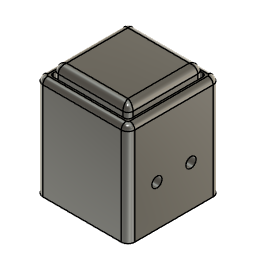
Z_LimitSwitchBox (Autodesk Fusion 360 design; units mm, degrees)
Autodesk Fusion 360 part; units mm, degrees
sketch "Sketch1" plane through (0, 0, 0) normal (0, 0, 1) x (1, 0, 0)
  line L0 (12.5, -12.5) -> (-12.5, -12.5)
  line L1 (-12.5, -12.5) -> (-12.5, 12.5)
  line L2 (-12.5, 12.5) -> (12.5, 12.5)
  line L3 (12.5, 12.5) -> (12.5, -12.5)
  line L4 (12.5, -12.5) -> (-12.5, 12.5) construction
  line L5 (-12.5, -12.5) -> (12.5, 12.5) construction
  line L6 (3.5, -10.5) -> (-3.5, -10.5)
  line L7 (-3.5, -10.5) -> (-3.5, 10.5)
  line L8 (-3.5, 10.5) -> (3.5, 10.5)
  line L9 (3.5, 10.5) -> (3.5, -10.5)
  line L10 (3.5, -10.5) -> (-3.5, 10.5) construction
  line L11 (-3.5, -10.5) -> (3.5, 10.5) construction
  line L12 (11.5, -11.5) -> (-11.5, -11.5)
  line L13 (-11.5, -11.5) -> (-11.5, 11.5)
  line L14 (-11.5, 11.5) -> (11.5, 11.5)
  line L15 (11.5, 11.5) -> (11.5, -11.5)
  line L16 (11.5, -11.5) -> (-11.5, 11.5) construction
  line L17 (-11.5, -11.5) -> (11.5, 11.5) construction
  dimension "d1" = 25
  dimension "d2" = 25
  dimension "d3" = 7
  dimension "d4" = 21
  dimension "d5" = 23
  dimension "d6" = 23
  constraint horizontal L0
  constraint perpendicular L0 L1
  constraint parallel L0 L2
  constraint parallel L1 L3
  constraint coincident L4 origin
  constraint coincident L5 origin
  constraint horizontal L6
  constraint perpendicular L6 L7
  constraint parallel L6 L8
  constraint parallel L7 L9
  constraint coincident L10 origin
  constraint coincident L11 origin
  constraint horizontal L12
  constraint perpendicular L12 L13
  constraint parallel L12 L14
  constraint parallel L13 L15
  constraint coincident L16 origin
  constraint coincident L17 origin
  measures "d1" distance of L1.end L2.end
  measures "d2" distance of L0.end L1.end
  measures "d3" distance of L7.end L8.end
  measures "d4" distance of L6.end L7.end
  measures "d5" distance of L13.end L14.end
  measures "d6" distance of L12.end L13.end
extrude "Extrude1" add sketch "Sketch1" along normal blind 30 contours L0 L1 L2 L3 | L6 L7 L8 L9 | L12 L13 L14 L15 makes body 1
extrude "Extrude2" cut sketch "Sketch1" along normal blind 1000 from surface at 5 contours L6 L7 L8 L9 bodies 1
extrude "Extrude3" cut sketch "Sketch1" along normal blind 100 from surface at 20 contours L12 L13 L14 L15 bodies 1
sketch "Sketch2" plane through (-12.5, 0, 0) normal (-1, 0, 0) x (0, -1, 0)
  line L0 (-12.5, 0) -> (12.5, 0)
  line L1 (12.5, 0) -> (12.5, 30)
  line L2 (12.5, 30) -> (-12.5, 30)
  line L3 (-12.5, 30) -> (-12.5, 0)
  line L4 (0, 12) -> (5, 12)
  line L5 (0, 12) -> (-5, 12)
  line L6 (-2.9, 13.2124) -> (-5, 14.4249)
  line L7 (-5, 14.4249) -> (-7.1, 13.2124)
  line L8 (-7.1, 13.2124) -> (-7.1, 10.7876)
  line L9 (-7.1, 10.7876) -> (-5, 9.5751)
  line L10 (-5, 9.5751) -> (-2.9, 10.7876)
  line L11 (-2.9, 10.7876) -> (-2.9, 13.2124)
  line L12 (7.1, 13.2124) -> (5, 14.4249)
  line L13 (5, 14.4249) -> (2.9, 13.2124)
  line L14 (2.9, 13.2124) -> (2.9, 10.7876)
  line L15 (2.9, 10.7876) -> (5, 9.5751)
  line L16 (5, 9.5751) -> (7.1, 10.7876)
  line L17 (7.1, 10.7876) -> (7.1, 13.2124)
  point P0 (-5, 12)
  point P1 (5, 12)
  dimension "d17" = 12
  dimension "d18" = 5
  dimension "d22" = 2.1
  dimension "d23" = 2.1
  constraint coincident P0 L5.end
  constraint coincident P1 L4.end
  measures "d17" distance of origin L4.start
  measures "d18" distance of L4.start P1
  measures "d22" distance of P0 L11
  measures "d23" distance of P1 L17
extrude "Extrude4" cut 1 faces at (1.1667, -3.5, 5) along direction (0, 0, -1) blind 2 on bodies 1 bodies 1
hole "Hole1" at (-12.5, -5, 12) at (-12.5, 5, 12) direction (1, 0, 0) diameter 3 depth 100 tip angle 118 bodies 1
extrude "Extrude5" cut sketch "Sketch2" against normal blind 1 contours L6 L7 L8 L9 L10 L11 | L12 L13 L14 L15 L16 L17 bodies 1
move_face "OffsetFaces1" offset 1 3 faces at (12.5, -1.5193, 24.4778) (-4.1667, 12.5, 20) (4.1667, -12.5, 20) on bodies 1
move_face "OffsetFaces2" offset 1 1 faces at (-12.5, 1.6667, 24.8083) on bodies 1
fillet "Fillet1" radius 2 4 edges at (-13.5, -13.5, 15) (13.5, -13.5, 15) (13.5, 13.5, 15) (-13.5, 13.5, 15) on bodies 1
fillet "Fillet2" radius 1 4 edges at (11.5, -11.5, 25) (11.5, 11.5, 25) (-11.5, 11.5, 25) (-11.5, -11.5, 25) on bodies 1
fillet "Fillet3" radius 1.5 8 edges at (12.9142, -12.9142, 30) (13.5, 0, 30) (12.9142, 12.9142, 30) (0, 13.5, 30) (-12.9142, 12.9142, 30) (-13.5, 0, 30) (-12.9142, -12.9142, 30) (0, -13.5, 30) on bodies 1
copy_body "Body->Comp1" bodies 1 removing the originals makes body 2 in component "Box1"
sketch "Sketch3" plane through (0, 0, 0) normal (0, 0, 1) x (1, 0, 0)
  line L0 (11, 11) -> (-11, 11)
  line L1 (-11, 11) -> (-11, -11)
  line L2 (-11, -11) -> (11, -11)
  line L3 (11, -11) -> (11, 11)
  line L4 (11, 11) -> (-11, -11) construction
  line L5 (-11, 11) -> (11, -11) construction
  dimension "d34" = 22
  dimension "d35" = 22
  constraint horizontal L0
  constraint perpendicular L0 L1
  constraint parallel L0 L2
  constraint parallel L1 L3
  constraint coincident L4 origin
  constraint coincident L5 origin
  measures "d34" distance of L1.end L2.end
  measures "d35" distance of L0.end L1.end
extrude "Extrude6" add sketch "Sketch3" along normal blind 13 separate body makes body 3
fillet "Fillet4" radius 1.5 4 edges at (11, -11, 6.5) (11, 11, 6.5) (-11, 11, 6.5) (-11, -11, 6.5) on bodies 3
fillet "Fillet5" radius 2 8 edges at (-11, 0, 13) (-10.5607, 10.5607, 13) (0, 11, 13) (10.5607, 10.5607, 13) (11, 0, 13) (10.5607, -10.5607, 13) (0, -11, 13) (-10.5607, -10.5607, 13) on bodies 3
copy_body "Body->Comp2" bodies 3 removing the originals makes body 4 in component "Plunger"
component "Box1" placed x (1, 0, 0) y (0, 1, 0) z (0, 0, 1) at (0, 0, 0)
component "Plunger" placed x (1, 0, 0) y (0, 1, 0) z (0, 0, 1) at (0, 0, 0)
